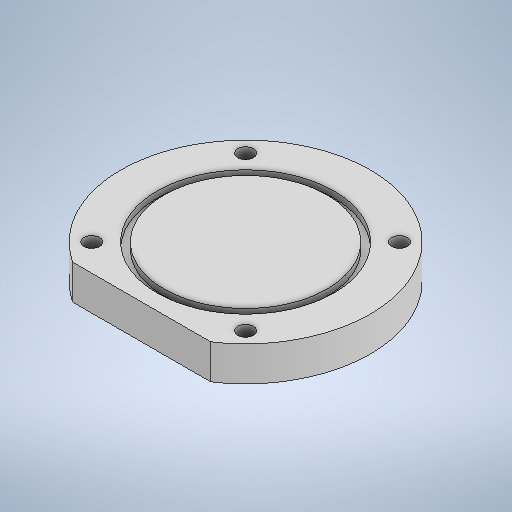
# Autodesk Inventor part: Access Cap
Saved by Autodesk Inventor 2025 (Build 290162000, 162)
## iProperties
Created: 2025-10-23
Part Number: Access Cap
Material: Generic
Document SubType Name: Modeling
Designer: mumin
Density: 1 g/cm^3
Appearance: Default
Author: mumin
Autodesk Inventor part; units mm, degrees
ref_plane "YZ Plane" through (0, 0, 0) normal (1, 0, 0) x (0, 1, 0)
ref_plane "XZ Plane" through (0, 0, 0) normal (0, 1, 0) x (-1, 0, 0)
ref_plane "XY Plane" through (0, 0, 0) normal (0, 0, 1) x (1, 0, 0)
sketch "Sketch1" plane through (0, 0, 0) normal (0, 1, 0) x (-1, 0, 0)
  circle A0 centre (0, 0) radius 36
  line L0 (19.8997, 30) -> (-19.8997, 30)
  dimension "d0" = 72
  dimension "d1" = 30
  constraints: 2 end point, 2 point on circle, 1 centre point, 1 coincident, 1 horizontal
  measures "d0" diameter of A0
  measures "d1" distance from line of point (0, 0) L0
extrude "Base" add sketch "Sketch1" along normal blind 10 contours A0 L0 picked at (-0.4083, 8.0069)
sketch "Sketch2" plane through (0, 0, 0) normal (0, -1, 0) x (1, 0, 0)
  circle A0 centre (0, 0) radius 31.4
  line L0 (22.2032, 22.2032) -> (0, 0)
  line L1 (-50.4, 0) -> (50.4, 0) projected
  dimension "d11" = 62.8
  dimension "d12" = 45
  constraints: 2 end point, 1 coincident, 3 other
  measures "d12" angle of L1 L0
hole "Mounting Holes" at (22.2032, 0, 22.2032) direction (0, 1, 0) diameter 4.5 end through all counterbore diameter 8 counterbore depth 4
pattern_circular "Circular Pattern1" count 4 over 360 about axis through (0, 0, 0) along (0, 1, 0) of "Mounting Holes"
sketch "Sketch3" plane through (0, 0, 0) normal (0, 0, 1) x (1, 0, 0)
  line L0 (36, 10) -> (-36, 10) projected
  line L1 (-25.5, 10) -> (-23.5, 10)
  line L2 (-23.5, 10) -> (-23.5, 8.2)
  line L3 (-23.5, 8.2) -> (-25.5, 8.2)
  line L4 (-25.5, 8.2) -> (-25.5, 10)
  line L5 (0, -2) -> (0, 12) projected
  point P0 (0, 0)
  point P1 (19.8997, 10)
  point P2 (-19.8997, 10)
  point P3 (0, 10)
  dimension "d16" = 2
  dimension "d17" = 1.8
  dimension "d18" = 23.5
  constraints: 8 end point, 2 parallel, 1 horizontal, 1 midpoint, 1 perpendicular, 1 point on line
  measures "d16" distance of L2.end L3.end
  measures "d17" distance of L1.end L2.end
  measures "d18" distance from line of point (0, 10) L2
revolve "Revolution1" cut sketch "Sketch3" angle 360 about axis through (0, -10, 0) along (0, 1, 0)
body "Solid1"
